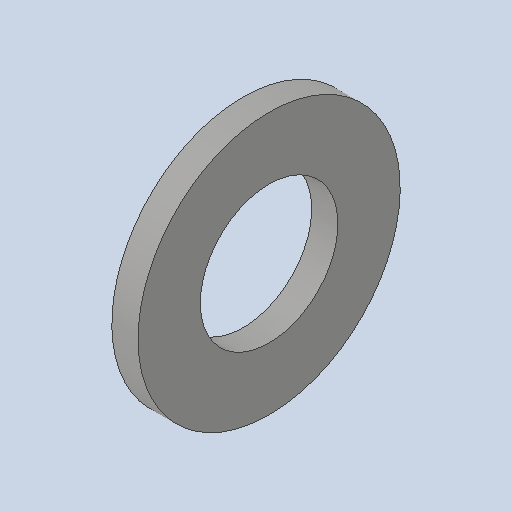
# Autodesk Inventor part: RobotunitsBLS_M008
Saved by Autodesk Inventor 2023 (Build 270158000, 158)
## iProperties
Created: 2023-08-22
Part Number: RobotunitsBLS_M008
Material: Generic
Catalog Web Link: www.cadenas.de
Description: BLS M008-Washer
Vendor: ROBOTUNITS
Document SubType Name: Modeling
Designer: psAdmin
Manufacturer: ROBOTUNITS
Mass: 0.233031 g
Surface Area: 4.13936 cm^2
Volume: 0.233031 cm^3
Density: 1 g/cm^3
Appearance: PSOLRGB-154-154-154
Category: PARTsolutions
Company: ROBOTUNITS
PSOL_IDENT_0: {$CADENAS_DATA/23d-libs/robotunits/profil_und_verbindungstechnik/verbindungstechnik_raster_40/parts/
PSOL_IDENT_1: bls_m008.prj},169 {VTYP=3D},{NB=RobotunitsBLS_M008},{LINA=RobotunitsBLS_M008},{NN=BLS M008},{DATE=01
PSOL_IDENT_2: .02.2021 08:30:02},{GEOMDATE=14.06.2007},{VERSION=},{LINEID=10},{WBVAR=},{WBNUMERIC=}  {NB=Robotunit
PSOL_IDENT_3: sBLS_M008},{LINA=RobotunitsBLS_M008},{KT=DUMMY},{ARTIKEL=BLS_M008}
NB: RobotunitsBLS_M008
NN: BLS M008
NT: Washer
NBSYN: Robotunits$ARTIKEL.
LINA: RobotunitsBLS_M008
CATALOG: Robotunits
ARTIKEL: BLS_M008
SUPPLIER: ROBOTUNITS
ARTICLENO: RobotunitsBLS_M008
BOMINFO: RobotunitsBLS_M008
CREATOR: CADENAS GmbH
Title: RobotunitsBLS_M008
Author: Cadenas PARTsolutions
Comments: Washer
Autodesk Inventor part; units mm, degrees
sketch "Skizze_1" plane through (0, 0, 0) normal (1, 0, 0) x (0, 1, 0)
  circle A0 centre (0, 0) radius 8
  circle A1 centre (0, 0) radius 4.2
  constraints: 2 centre point
extrude "Extrusion1" add sketch "Skizze_1" along normal blind 1.6
ref_plane "BLS_1_XY" through (0, 0, 0) normal (1, 0, 0) x (0, 0, -1)
ref_plane "BLS_1_YZ" through (0, 0, 0) normal (0, 0, -1) x (0, 1, 0)
ref_plane "BLS_1_ZX" through (0, 0, 0) normal (0, 1, 0) x (1, 0, 0)
body "Solid1"
